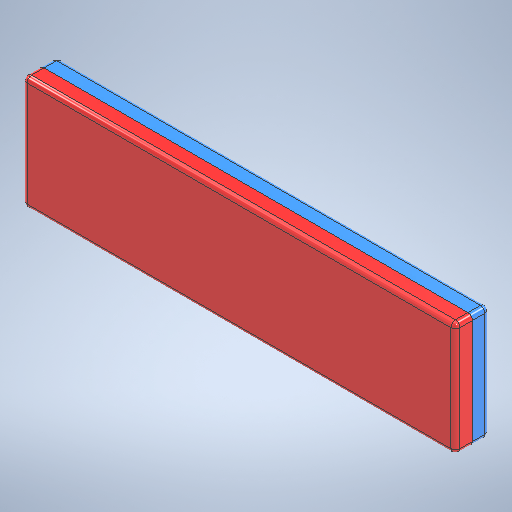
# Autodesk Inventor part: Magnet
Saved by Autodesk Inventor 2025 (Build 290162000, 162)
## iProperties
Created: 2025-03-06
Part Number: Magnet
Material: Generic
Document SubType Name: Modeling
Designer: tvoko
Density: 1 g/cm^3
Appearance: Default
Author: tvoko
Autodesk Inventor part; units mm, degrees
ref_plane "YZ Plane" through (0, 0, 0) normal (1, 0, 0) x (0, 1, 0)
ref_plane "XZ Plane" through (0, 0, 0) normal (0, 1, 0) x (-1, 0, 0)
sketch "Sketch1" plane through (0, 0, 0) normal (0, 1, 0) x (-1, 0, 0)
  line L0 (0, 0) -> (19, 0)
  line L1 (19, 0) -> (19, -1.5)
  line L2 (19, -1.5) -> (0, -1.5)
  line L3 (0, -1.5) -> (0, 0)
  dimension "d0" = 19
  dimension "d1" = 1.5
  constraints: 8 end point, 2 parallel, 1 horizontal, 1 perpendicular
  measures "d0" distance of L1.end L2.end
  measures "d1" distance of L0.end L1.end
extrude "Extrusion1" add sketch "Sketch1" along normal blind 5
fillet "Fillet1" radius 0.2 12 edges at (0, 2.5, 0) (0, 2.5, -1.5) (0, 0, -0.75) (0, 5, -0.75) (-19, 2.5, 0) (-9.5, 0, 0) (-9.5, 5, 0) (-19, 2.5, -1.5) (-19, 0, -0.75) (-19, 5, -0.75) (-9.5, 0, -1.5) (-9.5, 5, -1.5)
ref_plane "Work Plane1" through (-18.8, 0.2, -0.75) normal (0, 0, 1) x (1, 0, 0)
split body "Split1" result two bodies by plane through (-18.8, 0.2, -0.75) normal (0, 0, 1) first body at (-6.4, 1.6667, -0.25)
body "Solid2"
body "Solid3"
